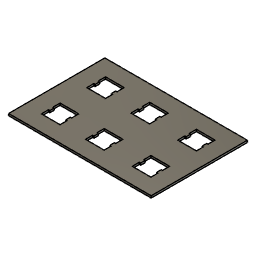
Taste_Halter_FULL v1 (Autodesk Fusion 360 design; units mm, degrees)
Autodesk Fusion 360 part; units mm, degrees
sketch "Skizze1" plane through (0, 0, 0) normal (0, 1, 0) x (1, 0, 0)
  line L0 (7, -7) -> (-7, -7)
  line L1 (-7, -7) -> (-7, 7)
  line L2 (-7, 7) -> (7, 7)
  line L3 (7, 7) -> (7, -7)
  line L4 (7, -7) -> (-7, 7) construction
  line L5 (-7, -7) -> (7, 7) construction
  line L6 (6, 1.65) -> (7, 1.65)
  line L7 (7, 1.65) -> (7, -1.65)
  line L8 (7, -1.65) -> (6, -1.65)
  line L9 (6, -1.65) -> (6, 1.65)
  line L10 (0, 0) -> (-0.0828, 0.0828)
  line L11 (0, 0) -> (0, 4.3114) construction
  line L12 (-7, -1.65) -> (-6, -1.65)
  line L13 (-6, -1.65) -> (-6, 1.65)
  line L14 (-7, 1.65) -> (-7, -1.65)
  line L15 (-6, 1.65) -> (-7, 1.65)
  line L16 (8, -8) -> (-8, -8) construction
  line L17 (-8, -8) -> (-8, 8) construction
  line L18 (-8, 8) -> (8, 8) construction
  line L19 (8, 8) -> (8, -8) construction
  line L20 (8, -8) -> (-8, 8) construction
  line L21 (-8, -8) -> (8, 8) construction
  line L22 (9, -9) -> (-9, -9)
  line L23 (-9, -9) -> (-9, 9)
  line L24 (-9, 9) -> (9, 9)
  line L25 (9, 9) -> (9, -9)
  line L26 (9, -9) -> (-9, 9) construction
  line L27 (-9, -9) -> (9, 9) construction
  line L28 (7, 7) -> (9, 7) construction
  line L29 (25, 8) -> (41, 8) construction
  line L30 (42, 9) -> (42, -9)
  line L31 (40, -7) -> (26, -7)
  line L32 (40, -7) -> (26, 7) construction
  line L33 (25, -8) -> (41, 8) construction
  line L34 (24, 9) -> (42, 9)
  line L35 (26, -7) -> (26, 7)
  line L36 (42, -9) -> (24, -9)
  line L37 (40, -1.65) -> (39, -1.65)
  line L38 (39, 1.65) -> (40, 1.65)
  line L39 (33, 0) -> (33, 4.3114) construction
  line L40 (39, -1.65) -> (39, 1.65)
  line L41 (40, 7) -> (40, -7)
  line L42 (33, 0) -> (32.9172, 0.0828)
  line L43 (40, 1.65) -> (40, -1.65)
  line L44 (41, 8) -> (41, -8) construction
  line L45 (25, -8) -> (25, 8) construction
  line L46 (40, 7) -> (42, 7) construction
  line L47 (27, -1.65) -> (27, 1.65)
  line L48 (41, -8) -> (25, 8) construction
  line L49 (41, -8) -> (25, -8) construction
  line L50 (26, -7) -> (40, 7) construction
  line L51 (26, 7) -> (40, 7)
  line L52 (42, -9) -> (24, 9) construction
  line L53 (26, 1.65) -> (26, -1.65)
  line L54 (26, -1.65) -> (27, -1.65)
  line L55 (24, -9) -> (24, 9)
  line L56 (27, 1.65) -> (26, 1.65)
  line L57 (24, -9) -> (42, 9) construction
  line L58 (33, -34) -> (33, -29.6886) construction
  line L59 (41, -42) -> (25, -26) construction
  line L60 (40, -41) -> (26, -27) construction
  line L61 (25, -42) -> (41, -26) construction
  line L62 (39, -35.65) -> (39, -32.35)
  line L63 (24, -43) -> (42, -25) construction
  line L64 (24, -25) -> (42, -25)
  line L65 (24, -43) -> (24, -25)
  line L66 (26, -41) -> (40, -27) construction
  line L67 (40, -27) -> (42, -27) construction
  line L68 (41, -26) -> (41, -42) construction
  line L69 (26, -32.35) -> (26, -35.65)
  line L70 (25, -42) -> (25, -26) construction
  line L71 (41, -42) -> (25, -42) construction
  line L72 (27, -35.65) -> (27, -32.35)
  line L73 (40, -35.65) -> (39, -35.65)
  line L74 (42, -43) -> (24, -43)
  line L75 (40, -41) -> (26, -41)
  line L76 (26, -41) -> (26, -27)
  line L77 (26, -35.65) -> (27, -35.65)
  line L78 (42, -43) -> (24, -25) construction
  line L79 (27, -32.35) -> (26, -32.35)
  line L80 (25, -26) -> (41, -26) construction
  line L81 (42, -25) -> (42, -43)
  line L82 (9, -43) -> (-9, -25) construction
  line L83 (8, -42) -> (-8, -42) construction
  line L84 (39, -32.35) -> (40, -32.35)
  line L85 (40, -32.35) -> (40, -35.65)
  line L86 (0, -34) -> (-0.0828, -33.9172)
  line L87 (-7, -35.65) -> (-6, -35.65)
  line L88 (8, -26) -> (8, -42) construction
  line L89 (6, -32.35) -> (7, -32.35)
  line L90 (0, -34) -> (0, -29.6886) construction
  line L91 (-9, -43) -> (9, -25) construction
  line L92 (7, -32.35) -> (7, -35.65)
  line L93 (7, -35.65) -> (6, -35.65)
  line L94 (7, -27) -> (7, -41)
  line L95 (6, -35.65) -> (6, -32.35)
  line L96 (-6, -32.35) -> (-7, -32.35)
  line L97 (-9, -43) -> (-9, -25)
  line L98 (9, -25) -> (9, -43)
  line L99 (-8, -26) -> (8, -26) construction
  line L100 (-8, -42) -> (-8, -26) construction
  line L101 (7, -41) -> (-7, -27) construction
  line L102 (-9, -25) -> (9, -25)
  line L103 (7, -27) -> (9, -27) construction
  line L104 (-7, -41) -> (-7, -27)
  line L105 (8, -42) -> (-8, -26) construction
  line L106 (-7, -32.35) -> (-7, -35.65)
  line L107 (-7, -27) -> (7, -27)
  line L108 (-6, -35.65) -> (-6, -32.35)
  line L109 (7, -41) -> (-7, -41)
  line L110 (-8, -42) -> (8, -26) construction
  line L111 (-7, -41) -> (7, -27) construction
  line L112 (9, -43) -> (-9, -43)
  line L113 (33, -34) -> (32.9172, -33.9172)
  line L114 (40, -27) -> (40, -41)
  line L115 (26, -27) -> (40, -27)
  line L116 (68, -34) -> (67.9172, -33.9172)
  line L117 (60, -42) -> (60, -26) construction
  line L118 (61, -41) -> (61, -27)
  line L119 (61, -35.65) -> (62, -35.65)
  line L120 (62, -32.35) -> (61, -32.35)
  line L121 (61, -32.35) -> (61, -35.65)
  line L122 (68, -34) -> (68, -29.6886) construction
  line L123 (61, -7) -> (61, 7)
  line L124 (62, -35.65) -> (62, -32.35)
  line L125 (59, -43) -> (59, -25)
  line L126 (68, 0) -> (68, 4.3114) construction
  line L127 (68, 0) -> (67.9172, 0.0828)
  line L128 (61, -7) -> (75, 7) construction
  line L129 (59, -9) -> (59, 9)
  line L130 (62, -1.65) -> (62, 1.65)
  line L131 (61, -1.65) -> (62, -1.65)
  line L132 (75, -7) -> (61, 7) construction
  line L133 (62, 1.65) -> (61, 1.65)
  line L134 (61, 1.65) -> (61, -1.65)
  line L135 (60, -8) -> (60, 8) construction
  line L136 (77, -25) -> (77, -43)
  line L137 (74, -32.35) -> (75, -32.35)
  line L138 (77, -9) -> (59, 9) construction
  line L139 (75, -32.35) -> (75, -35.65)
  line L140 (75, -35.65) -> (74, -35.65)
  line L141 (75, -27) -> (75, -41)
  line L142 (76, -26) -> (76, -42) construction
  line L143 (76, -8) -> (60, 8) construction
  line L144 (74, -35.65) -> (74, -32.35)
  line L145 (75, -27) -> (77, -27) construction
  line L146 (59, -9) -> (77, 9) construction
  line L147 (74, 1.65) -> (75, 1.65)
  line L148 (60, -8) -> (76, 8) construction
  line L149 (76, -8) -> (60, -8) construction
  line L150 (60, -26) -> (76, -26) construction
  line L151 (75, -41) -> (61, -41)
  line L152 (61, -27) -> (75, -27)
  line L153 (60, -42) -> (76, -26) construction
  line L154 (76, -42) -> (60, -26) construction
  line L155 (77, -9) -> (59, -9)
  line L156 (75, 7) -> (77, 7) construction
  line L157 (59, 9) -> (77, 9)
  line L158 (76, 8) -> (76, -8) construction
  line L159 (59, -25) -> (77, -25)
  line L160 (75, 1.65) -> (75, -1.65)
  line L161 (61, -41) -> (75, -27) construction
  line L162 (77, 9) -> (77, -9)
  line L163 (76, -42) -> (60, -42) construction
  line L164 (60, 8) -> (76, 8) construction
  line L165 (77, -43) -> (59, -25) construction
  line L166 (75, -1.65) -> (74, -1.65)
  line L167 (75, -41) -> (61, -27) construction
  line L168 (59, -43) -> (77, -25) construction
  line L169 (77, -43) -> (59, -43)
  line L170 (61, 7) -> (75, 7)
  line L171 (75, 7) -> (75, -7)
  line L172 (74, -1.65) -> (74, 1.65)
  line L173 (75, -7) -> (61, -7)
  line L174 (-9, -9) -> (77, -9)
  line L175 (77, -9) -> (77, -25)
  line L176 (77, -25) -> (-9, -25)
  line L177 (-9, -25) -> (-9, -9)
  line L178 (42, 9) -> (59, 9)
  line L179 (59, 9) -> (59, -9)
  line L180 (59, -9) -> (42, -9)
  line L181 (42, -9) -> (42, 9)
  line L182 (9, 9) -> (24, 9)
  line L183 (24, 9) -> (24, -9)
  line L184 (24, -9) -> (9, -9)
  line L185 (9, -9) -> (9, 9)
  line L186 (9, -25) -> (24, -25)
  line L187 (24, -25) -> (24, -43)
  line L188 (24, -43) -> (9, -43)
  line L189 (9, -43) -> (9, -25)
  line L190 (42, -25) -> (59, -25)
  line L191 (59, -25) -> (59, -43)
  line L192 (59, -43) -> (42, -43)
  line L193 (42, -43) -> (42, -25)
  line L194 (-9, -43) -> (77, -43)
  line L195 (77, -43) -> (77, -53)
  line L196 (77, -53) -> (-9, -53)
  line L197 (-9, -53) -> (-9, -43)
  line L198 (77, 9) -> (-9, 9)
  line L199 (-9, 9) -> (-9, 19)
  line L200 (-9, 19) -> (77, 19)
  line L201 (77, 19) -> (77, 9)
  line L202 (77, 19) -> (77, 19)
  line L203 (77, 19) -> (77, -53)
  line L204 (77, -53) -> (77, -53)
  line L205 (77, -53) -> (77, 19)
  line L206 (77, -53) -> (87.1689, -53)
  line L207 (87.1689, -53) -> (87.1689, 19)
  line L208 (87.1689, 19) -> (77, 19)
  line L209 (77, 19) -> (77, -53)
  line L210 (-9, -53) -> (-19.4967, -53)
  line L211 (-19.4967, -53) -> (-19.4967, 19)
  line L212 (-19.4967, 19) -> (-9, 19)
  line L213 (-9, 19) -> (-9, -53)
  point P0 (33, 0)
  point P1 (33, 0)
  point P2 (33, 0)
  point P3 (0, -34)
  point P4 (0, -34)
  point P5 (0, -34)
  point P6 (33, -34)
  point P7 (33, -34)
  point P8 (33, -34)
  point P9 (68, 0)
  point P10 (68, 0)
  point P11 (68, 0)
  point P12 (68, -34)
  point P13 (68, -34)
  point P14 (68, -34)
  dimension "d1" = 14
  dimension "d2" = 14
  dimension "d6" = 1
  dimension "d7" = 3.3
  dimension "d8" = 16
  dimension "d9" = 16
  dimension "d10" = 18
  dimension "d11" = 18
  dimension "d13" = 2
  dimension "d19" = 14
  dimension "d20" = 14
  dimension "d21" = 1
  dimension "d22" = 3.3
  dimension "d23" = 16
  dimension "d24" = 16
  dimension "d25" = 18
  dimension "d26" = 18
  dimension "d27" = 2
  dimension "d28" = 14
  dimension "d29" = 14
  dimension "d30" = 1
  dimension "d31" = 3.3
  dimension "d32" = 16
  dimension "d33" = 16
  dimension "d34" = 18
  dimension "d35" = 18
  dimension "d36" = 2
  dimension "d37" = 14
  dimension "d38" = 14
  dimension "d39" = 1
  dimension "d40" = 3.3
  dimension "d41" = 16
  dimension "d42" = 16
  dimension "d43" = 18
  dimension "d44" = 18
  dimension "d45" = 2
  dimension "d46" = 14
  dimension "d47" = 14
  dimension "d48" = 1
  dimension "d49" = 3.3
  dimension "d50" = 16
  dimension "d51" = 16
  dimension "d52" = 18
  dimension "d53" = 18
  dimension "d54" = 2
  dimension "d55" = 14
  dimension "d56" = 14
  dimension "d57" = 1
  dimension "d58" = 3.3
  dimension "d59" = 16
  dimension "d60" = 16
  dimension "d61" = 18
  dimension "d62" = 18
  dimension "d63" = 2
  constraint horizontal L0
  constraint perpendicular L0 L1
  constraint parallel L0 L2
  constraint parallel L1 L3
  constraint coincident L4 L10.start
  constraint coincident L5 L10.start
  constraint coincident L10.start L11.start
  constraint horizontal L6
  constraint vertical L7
  constraint horizontal L8
  constraint vertical L9
  constraint midpoint L3 L7
  constraint coincident L4 L10.end
  constraint parallel L4 L10
  constraint vertical L11
  constraint symmetric L6.start L11 L13.end
  constraint symmetric L6.end L11 L14.start
  constraint symmetric L7.end L11 L12.start
  constraint symmetric L8.end L11 L12.end
  constraint horizontal L16
  constraint perpendicular L16 L17
  constraint parallel L16 L18
  constraint parallel L17 L19
  constraint coincident L20 L10.start
  constraint coincident L21 L10.start
  constraint horizontal L22
  constraint perpendicular L22 L23
  constraint parallel L22 L24
  constraint parallel L23 L25
  constraint coincident L26 L10.start
  constraint coincident L27 L10.start
  constraint coincident L25 L28.end
  constraint perpendicular L25 L28
  constraint horizontal L31
  constraint perpendicular L31 L35
  constraint parallel L31 L51
  constraint parallel L35 L41
  constraint coincident P2 L32
  constraint coincident P2 L50
  constraint horizontal L38
  constraint vertical L43
  constraint horizontal L37
  constraint vertical L40
  constraint midpoint L41 L43
  constraint coincident P2 P1
  constraint coincident L42.end L32
  constraint parallel L32 L42
  constraint vertical L39
  constraint symmetric L38.start L47.end L39
  constraint symmetric L38.end L53.start L39
  constraint symmetric L53.end L37.start L39
  constraint symmetric L37.end L47.start L39
  constraint horizontal L49
  constraint perpendicular L45 L49
  constraint parallel L29 L49
  constraint parallel L44 L45
  constraint coincident P2 L48
  constraint coincident P2 L33
  constraint horizontal L36
  constraint perpendicular L36 L55
  constraint parallel L34 L36
  constraint parallel L30 L55
  constraint coincident P2 L52
  constraint coincident P2 L57
  constraint coincident L46.end L30
  constraint perpendicular L30 L46
  constraint horizontal L109
  constraint perpendicular L104 L109
  constraint parallel L107 L109
  constraint parallel L94 L104
  constraint coincident P5 L101
  constraint coincident P5 L111
  constraint horizontal L89
  constraint vertical L92
  constraint horizontal L93
  constraint vertical L95
  constraint midpoint L92 L94
  constraint coincident P5 P4
  constraint coincident L86.end L101
  constraint parallel L86 L101
  constraint vertical L90
  constraint symmetric L89.start L96.start L90
  constraint symmetric L89.end L96.end L90
  constraint symmetric L87.start L92.end L90
  constraint symmetric L93.end L87.end L90
  constraint horizontal L83
  constraint perpendicular L83 L100
  constraint parallel L83 L99
  constraint parallel L88 L100
  constraint coincident P5 L105
  constraint coincident P5 L110
  constraint horizontal L112
  constraint perpendicular L97 L112
  constraint parallel L102 L112
  constraint parallel L97 L98
  constraint coincident P5 L82
  constraint coincident P5 L91
  constraint coincident L103.end L98
  constraint perpendicular L98 L103
  constraint horizontal L75
  constraint perpendicular L75 L76
  constraint parallel L75 L115
  constraint parallel L76 L114
  constraint coincident P8 L60
  constraint coincident P8 L66
  constraint horizontal L84
  constraint vertical L85
  constraint horizontal L73
  constraint vertical L62
  constraint midpoint L85 L114
  constraint coincident P8 P7
  constraint coincident L113.end L60
  constraint parallel L60 L113
  constraint vertical L58
  constraint symmetric L72.end L62.end L58
  constraint symmetric L84.end L69.start L58
  constraint symmetric L69.end L73.start L58
  constraint symmetric L62.start L72.start L58
  constraint horizontal L71
  constraint perpendicular L70 L71
  constraint parallel L71 L80
  constraint parallel L68 L70
  constraint coincident P8 L59
  constraint coincident P8 L61
  constraint horizontal L74
  constraint perpendicular L65 L74
  constraint parallel L64 L74
  constraint parallel L65 L81
  constraint coincident P8 L78
  constraint coincident P8 L63
  constraint coincident L67.end L81
  constraint perpendicular L67 L81
  constraint horizontal L173
  constraint perpendicular L123 L173
  constraint parallel L170 L173
  constraint parallel L123 L171
  constraint coincident P11 L132
  constraint coincident P11 L128
  constraint horizontal L147
  constraint vertical L160
  constraint horizontal L166
  constraint vertical L172
  constraint midpoint L160 L171
  constraint coincident P11 P10
  constraint coincident L127.end L132
  constraint parallel L127 L132
  constraint vertical L126
  constraint symmetric L130.end L147.start L126
  constraint symmetric L147.end L133.end L126
  constraint symmetric L131.start L160.end L126
  constraint symmetric L166.end L130.start L126
  constraint horizontal L149
  constraint perpendicular L135 L149
  constraint parallel L149 L164
  constraint parallel L135 L158
  constraint coincident P11 L143
  constraint coincident P11 L148
  constraint horizontal L155
  constraint perpendicular L129 L155
  constraint parallel L155 L157
  constraint parallel L129 L162
  constraint coincident P11 L138
  constraint coincident P11 L146
  constraint coincident L156.end L162
  constraint perpendicular L156 L162
  constraint horizontal L151
  constraint perpendicular L118 L151
  constraint parallel L151 L152
  constraint parallel L118 L141
  constraint coincident P14 L167
  constraint coincident P14 L161
  constraint horizontal L137
  constraint vertical L139
  constraint horizontal L140
  constraint vertical L144
  constraint midpoint L139 L141
  constraint coincident P14 P13
  constraint coincident L116.end L167
  constraint parallel L116 L167
  constraint vertical L122
  constraint symmetric L137.start L120.start L122
  constraint symmetric L137.end L120.end L122
  constraint symmetric L119.start L139.end L122
  constraint symmetric L119.end L140.end L122
  constraint horizontal L163
  constraint perpendicular L117 L163
  constraint parallel L150 L163
  constraint parallel L117 L142
  constraint coincident P14 L154
  constraint coincident P14 L153
  constraint horizontal L169
  constraint perpendicular L125 L169
  constraint parallel L159 L169
  constraint parallel L125 L136
  constraint coincident P14 L165
  constraint coincident P14 L168
  constraint coincident L145.end L136
  constraint perpendicular L136 L145
  constraint horizontal L174
  constraint vertical L175
  constraint horizontal L176
  constraint vertical L177
  constraint horizontal L178
  constraint vertical L179
  constraint horizontal L180
  constraint vertical L181
  constraint horizontal L182
  constraint vertical L183
  constraint horizontal L184
  constraint vertical L185
  constraint horizontal L186
  constraint vertical L187
  constraint horizontal L188
  constraint vertical L189
  constraint horizontal L190
  constraint vertical L191
  constraint horizontal L192
  constraint vertical L193
  constraint horizontal L194
  constraint vertical L195
  constraint horizontal L196
  constraint vertical L197
  constraint horizontal L198
  constraint vertical L199
  constraint horizontal L200
  constraint vertical L201
  constraint vertical L203
  constraint vertical L205
  constraint horizontal L206
  constraint vertical L207
  constraint horizontal L208
  constraint vertical L209
  constraint horizontal L210
  constraint vertical L211
  constraint horizontal L212
  constraint vertical L213
  measures "d1" distance of L1.end L2.end
  measures "d2" distance of L0.end L1.end
  measures "d6" distance of L6.start L6.end
  measures "d7" distance of L6.start L8.end
  measures "d8" distance of L17.end L18.end
  measures "d9" distance of L16.end L17.end
  measures "d10" distance of L23.end L24.end
  measures "d11" distance of L22.end L23.end
  measures "d13" distance of L2.end L28.end
  measures "d19" distance of L32.end L41.start
  measures "d20" distance of L32.end L31.end
  measures "d21" distance of L38.end L38.start
  measures "d22" distance of L38.start L37.end
  measures "d23" distance of L29.start L29.end
  measures "d24" distance of L33.start L29.start
  measures "d25" distance of L34.start L30.start
  measures "d26" distance of L36.end L34.start
  measures "d27" distance of L41.start L46.end
  measures "d28" distance of L101.end L94.start
  measures "d29" distance of L101.end L104.start
  measures "d30" distance of L89.end L89.start
  measures "d31" distance of L89.start L93.end
  measures "d32" distance of L99.start L88.start
  measures "d33" distance of L83.end L99.start
  measures "d34" distance of L82.end L91.end
  measures "d35" distance of L91.start L82.end
  measures "d36" distance of L94.start L103.end
  measures "d37" distance of L66.end L60.end
  measures "d38" distance of L60.end L66.start
  measures "d39" distance of L84.end L62.end
  measures "d40" distance of L62.start L62.end
  measures "d41" distance of L61.end L59.end
  measures "d42" distance of L61.start L59.end
  measures "d43" distance of L64.start L63.end
  measures "d44" distance of L64.start L63.start
  measures "d45" distance of L66.end L67.end
  measures "d46" distance of L128.end L123.end
  measures "d47" distance of L123.end L123.start
  measures "d48" distance of L147.end L147.start
  measures "d49" distance of L166.end L147.start
  measures "d50" distance of L148.end L135.end
  measures "d51" distance of L135.start L135.end
  measures "d52" distance of L129.end L146.end
  measures "d53" distance of L129.end L129.start
  measures "d54" distance of L128.end L156.end
  measures "d55" distance of L118.end L141.start
  measures "d56" distance of L118.end L118.start
  measures "d57" distance of L137.end L137.start
  measures "d58" distance of L137.start L140.end
  measures "d59" distance of L142.start L117.end
  measures "d60" distance of L117.start L117.end
  measures "d61" distance of L136.start L125.end
  measures "d62" distance of L125.end L125.start
  measures "d63" distance of L141.start L145.end
extrude "Extrusion2" add sketch "Skizze1" along normal blind 1.5 contours L3 L6 L7 L8 L9 | L1 L12 L13 L14 L15 | L22 L36 L64 L102 L155 L159 L174 L175 L176 L177 L180 L184 L186 L190 L203 L205 L209 L213 | L22 L23 L24 L25 L174 L185 L198 L213 | L25 L55 L174 L182 L183 L184 L185 L198 | L23 L97 L177 L197 L199 L210 L211 L212 L213 | L24 L34 L157 L178 L182 L198 L199 L200 L201 L203 L205 L209 L213 | L30 L34 L36 L55 L174 L181 L183 L198 | L97 L98 L102 L112 L176 L189 L194 L213 | L30 L129 L174 L178 L179 L180 L181 L198 | L74 L112 L169 L188 L192 L194 L195 L196 L197 L203 L205 L209 L213 | L65 L98 L176 L186 L187 L188 L189 L194 | L129 L155 L157 L162 L174 L179 L198 L203 L205 L209 | L136 L162 L175 L195 L201 L203 L205 L206 L207 L208 L209 | L64 L65 L74 L81 L176 L187 L193 L194 | L81 L125 L176 L190 L191 L192 L193 L194 | L125 L136 L159 L169 L176 L191 L194 L203 L205 L209 | L37 L38 L40 L41 L43 | L35 L47 L53 L54 L56 | L62 L73 L84 L85 L114 | L69 L72 L76 L77 L79 | L87 L96 L104 L106 L108 | L89 L92 L93 L94 L95 | L118 L119 L120 L121 L124 | L137 L139 L140 L141 L144 | L123 L130 L131 L133 L134 | L147 L160 L166 L171 L172
extrude "Extrusion1" [suppressed]
chamfer "Fase1" [suppressed]
equation "d11 = d10"
equation "d26 = d10"
equation "d35 = d10"
equation "d44 = d10"
equation "d53 = d10"
equation "d62 = d10"
named bodies: "tasthalter2"
